1-5-000 PC_v2 (Autodesk Fusion 360 design; units mm, degrees)
Autodesk Fusion 360 part; units mm, degrees
sketch "Sketch1" plane through (0, 0, 0) normal (0, 0, 1) x (1, 0, 0) in component "PC"
  line L0 (206.375, 107.95) -> (-206.375, 107.95)
  line L1 (-206.375, 107.95) -> (-206.375, -107.95)
  line L2 (-206.375, -107.95) -> (206.375, -107.95)
  line L3 (206.375, -107.95) -> (206.375, 107.95)
  line L4 (206.375, 107.95) -> (-206.375, -107.95) construction
  line L5 (-206.375, 107.95) -> (206.375, -107.95) construction
  dimension "d1" = 412.75
  dimension "d2" = 215.9
  constraint horizontal L0
  constraint perpendicular L0 L1
  constraint parallel L0 L2
  constraint parallel L1 L3
  constraint coincident L4 origin
  constraint coincident L5 origin
  measures "d1" distance of L1.end L2.end
  measures "d2" distance of L0.end L1.end
extrude "Extrude1" add sketch "Sketch1" along normal blind 463.55 in component "PC"
component "PC" placed x (1, 0, 0) y (0, 1, 0) z (0, 0, 1) at (0, 0, 0)
